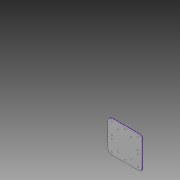
# Autodesk Inventor part: J1_Base
Saved by Autodesk Inventor 2020 (Build 240168000, 168)
## iProperties
Created: 2021-03-23
Part Number: J1_Base
Material: Generic
Document SubType Name: Modeling
Designer: DDeGo
Density: 1 g/cm^3
Appearance: Default
Author: DDeGo
Autodesk Inventor part; units mm, degrees
ref_plane "YZ Plane" through (0, 0, 0) normal (1, 0, 0) x (0, 1, 0)
ref_plane "XZ Plane" through (0, 0, 0) normal (0, 1, 0) x (-1, 0, 0)
ref_plane "XY Plane" through (0, 0, 0) normal (0, 0, 1) x (1, 0, 0)
sketch "Block1" plane through (0, 0, 0) normal (0, 0, 1) x (1, 0, 0)
  circle A0 centre (104.3747, 98.902) radius 2.75
  line L0 (74.8497, 87.402) -> (74.8497, 42.402) construction
  circle A1 centre (67.3497, 52.402) radius 2.75
  line L1 (59.8497, 42.402) -> (59.8497, 122.902) construction
  line L2 (59.8497, 42.402) -> (74.8497, 42.402) construction
  arc A2 (79.8497, 92.402) -> (74.8497, 87.402) centre (79.8497, 87.402) ccw construction
  circle A3 centre (66.3497, 118.402) radius 2.75
  line L3 (59.8497, 122.902) -> (61.8497, 124.902) construction
  line L4 (79.8497, 92.402) -> (204.9497, 92.402) construction
  line L5 (61.8497, 124.902) -> (222.9497, 124.902) construction
  circle A4 centre (142.3997, 118.402) radius 2.75
  circle A5 centre (180.4247, 98.902) radius 2.75
  arc A6 (209.9497, 87.402) -> (204.9497, 92.402) centre (204.9497, 87.402) ccw construction
  circle A7 centre (218.4497, 118.402) radius 2.75
  line L6 (222.9497, 124.902) -> (224.9497, 122.902) construction
  line L7 (209.9497, 87.402) -> (209.9497, 42.402) construction
  line L8 (224.9497, 42.402) -> (224.9497, 122.902) construction
  circle A8 centre (217.4497, 52.402) radius 2.75
  line L9 (224.9497, 42.402) -> (209.9497, 42.402) construction
  point P0 (142.3997, 87.8737)
  point P1 (142.3997, 92.402)
sketch "Sketch1" plane through (0, 0, 0) normal (0, 0, 1) x (1, 0, 0)
  line L0 (77.5, -90) -> (-77.5, -90)
  line L1 (-97.5, -70) -> (-97.5, 70)
  line L2 (-77.5, 90) -> (77.5, 90)
  line L3 (97.5, 70) -> (97.5, -70)
  line L4 (97.5, -90) -> (-97.5, 90) construction
  line L5 (-97.5, -90) -> (97.5, 90) construction
  arc A0 (-77.5, 90) -> (-97.5, 70) centre (-77.5, 70) ccw
  arc A1 (97.5, 70) -> (77.5, 90) centre (77.5, 70) ccw
  arc A2 (77.5, -90) -> (97.5, -70) centre (77.5, -70) ccw
  arc A3 (-97.5, -70) -> (-77.5, -90) centre (-77.5, -70) ccw
  point P0 (0, 0)
  dimension "d1" = 195
  dimension "d2" = 180
  dimension "d3" = 20
  constraints: 12 end point, 8 point on circle, 8 point on line, 8 tangent, 4 centre point, 3 equal radius, 2 midpoint, 2 parallel, 1 horizontal, 1 perpendicular
  measures "d1" distance between parallel lines of L3 L1
  measures "d2" distance between parallel lines of L0 L2
  measures "d3" radius of A0
extrude "Extrusion1" add sketch "Sketch1" along normal blind 6
sketch "Sketch2" plane through (0, 0, 6) normal (0, 0, 1) x (1, 0, 0)
  line L0 (0, 0) -> (-97.5, 0) construction
  line L1 (-97.5, 70) -> (-97.5, -70) projected
  line L2 (0, 0) -> (0, 52.5) construction
  circle A0 centre (-38.025, 59) radius 2.75
  line L3 (-67.55, 47.5) -> (-67.55, 2.5) construction
  circle A1 centre (-75.05, 12.5) radius 2.75
  line L4 (-82.55, 2.5) -> (-82.55, 83) construction
  line L5 (-82.55, 2.5) -> (-67.55, 2.5) construction
  arc A2 (-62.55, 52.5) -> (-67.55, 47.5) centre (-62.55, 47.5) ccw construction
  circle A3 centre (-76.05, 78.5) radius 2.75
  line L6 (-82.55, 83) -> (-80.55, 85) construction
  line L7 (-62.55, 52.5) -> (62.55, 52.5) construction
  line L8 (-80.55, 85) -> (80.55, 85) construction
  circle A4 centre (0, 78.5) radius 2.75
  circle A5 centre (38.025, 59) radius 2.75
  arc A6 (67.55, 47.5) -> (62.55, 52.5) centre (62.55, 47.5) ccw construction
  circle A7 centre (76.05, 78.5) radius 2.75
  line L9 (80.55, 85) -> (82.55, 83) construction
  line L10 (67.55, 47.5) -> (67.55, 2.5) construction
  line L11 (82.55, 2.5) -> (82.55, 83) construction
  circle A8 centre (75.05, 12.5) radius 2.75
  line L12 (82.55, 2.5) -> (67.55, 2.5) construction
  circle A9 centre (-38.025, -59) radius 2.75
  line L13 (-67.55, -47.5) -> (-67.55, -2.5) construction
  circle A10 centre (-75.05, -12.5) radius 2.75
  line L14 (-82.55, -2.5) -> (-82.55, -83) construction
  line L15 (-82.55, -2.5) -> (-67.55, -2.5) construction
  arc A11 (-62.55, -52.5) -> (-67.55, -47.5) centre (-62.55, -47.5) cw construction
  circle A12 centre (-76.05, -78.5) radius 2.75
  line L16 (-82.55, -83) -> (-80.55, -85) construction
  line L17 (-62.55, -52.5) -> (62.55, -52.5) construction
  line L18 (-80.55, -85) -> (80.55, -85) construction
  circle A13 centre (0, -78.5) radius 2.75
  circle A14 centre (38.025, -59) radius 2.75
  arc A15 (67.55, -47.5) -> (62.55, -52.5) centre (62.55, -47.5) cw construction
  circle A16 centre (76.05, -78.5) radius 2.75
  line L19 (80.55, -85) -> (82.55, -83) construction
  line L20 (67.55, -47.5) -> (67.55, -2.5) construction
  line L21 (82.55, -2.5) -> (82.55, -83) construction
  circle A17 centre (75.05, -12.5) radius 2.75
  line L22 (82.55, -2.5) -> (67.55, -2.5) construction
  dimension "d6" = 52.5
  constraints: 4 end point, 1 horizontal, 1 midpoint, 1 vertical, 1 other
  measures "d6" distance of L0.start L2.end
extrude "Extrusion2" cut sketch "Sketch2" against normal through all
body "Solid1"
